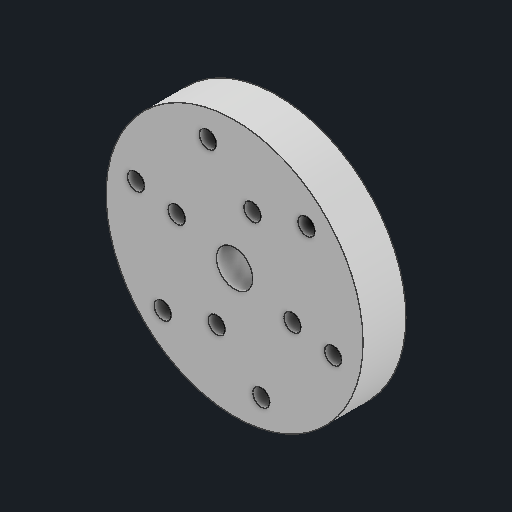
# Autodesk Inventor part: LegHub
Saved by Autodesk Inventor 2025.2 (Build 292293000, 293)
## iProperties
Created: 2025-10-06
Part Number: LegHub
Material: Generic
Document SubType Name: Modeling
Designer: valer
Density: 1 g/cm^3
Appearance: Default
Author: valer
Autodesk Inventor part; units mm, degrees
ref_plane "YZ Plane" through (0, 0, 0) normal (1, 0, 0) x (0, 1, 0)
ref_plane "XZ Plane" through (0, 0, 0) normal (0, 1, 0) x (-1, 0, 0)
ref_plane "XY Plane" through (0, 0, 0) normal (0, 0, 1) x (1, 0, 0)
sketch "Sketch1" plane through (0, 0, 0) normal (0, 0, 1) x (1, 0, 0)
  circle A0 centre (0, 0) radius 30
  dimension "d0" = 60
  constraints: 1 centre point, 1 coincident
  measures "d0" diameter of A0
extrude "Extrusion1" add sketch "Sketch1" along normal blind 10
sketch "Sketch2" plane through (0, 0, 10) normal (0, 0, 1) x (1, 0, 0)
  circle A0 centre (6.2371, -22.9812) radius 1.9939
  circle A1 centre (23.0208, -6.0891) radius 1.9939
  circle A2 centre (-23.0208, 6.0891) radius 1.9939
  circle A3 centre (-16.7837, -16.8921) radius 1.9939
  circle A4 centre (-6.2371, 22.9812) radius 1.9939
  circle A5 centre (16.7837, 16.8921) radius 1.9939
  circle A6 centre (0, 0) radius 14.2875 construction
  point P0 (0, 0)
extrude "Extrusion2" cut sketch "Sketch2" against normal through all
sketch "Sketch3" plane through (0, 0, 0) normal (0, 0, -1) x (-1, 0, 0)
  circle A0 centre (-13.511, -4.1777) radius 2 projected
  circle A1 centre (-4.1777, 13.511) radius 2 projected
  circle A2 centre (4.1777, -13.511) radius 2 projected
  circle A3 centre (13.511, 4.1777) radius 2 projected
  circle A4 centre (4.1777, -13.511) radius 2 projected
  point P0 (0, 0)
extrude "Extrusion3" cut sketch "Sketch3" against normal through all
sketch "Sketch4" plane through (0, 0, 0) normal (0, 0, -1) x (-1, 0, 0)
  circle A0 centre (0, 0) radius 4 construction
  circle A1 centre (-4.1777, 13.511) radius 2 projected
  circle A2 centre (13.511, 4.1777) radius 2 projected
  circle A3 centre (-13.511, -4.1777) radius 2 projected
  circle A4 centre (4.1777, -13.511) radius 2 projected
  circle A5 centre (-6.2371, -22.9812) radius 1.9939 projected
  circle A6 centre (6.2371, 22.9812) radius 1.9939 projected
  circle A7 centre (-23.0208, -6.0891) radius 1.9939 projected
  circle A8 centre (16.7837, -16.8921) radius 1.9939 projected
  circle A9 centre (23.0208, 6.0891) radius 1.9939 projected
  circle A10 centre (-16.7837, 16.8921) radius 1.9939 projected
  circle A11 centre (0, 0) radius 30 projected
  circle A12 centre (0, 0) radius 4.25
  dimension "d7" = 8.5
  constraints: 1 centre point, 1 coincident
  measures "d7" diameter of A12
extrude "Extrusion4" cut sketch "Sketch4" against normal through all contours A12
sketch "Sketch5" plane through (0, 0, 0) normal (0, 0, -1) x (-1, 0, 0)
  circle A0 centre (0, 0) radius 12.25 construction
  circle A1 centre (0, 0) radius 4.25 projected
  circle A2 centre (0, 0) radius 12
  dimension "d10" = 24
  constraints: 1 centre point, 1 coincident
  measures "d10" diameter of A2
body "Solid1"
